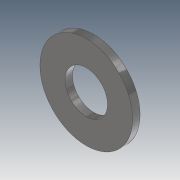
# Autodesk Inventor part: MCMASTER 92141A009
Saved by Autodesk Inventor 2020.4 (Build 244396000, 396)
## iProperties
RuleStatus: InUse
AfterDocSave0: file://Part Number Cleaner
Created: 2014-07-21
Material: STAINLESS STEEL, 18-8
Vendor: HHMI: JFRC - ID&F
Document SubType Name: Modeling
Designer: COOPB
Mass: 0.342993 g
Surface Area: 1.45791 cm^2
Volume: 0.0428742 cm^3
Density: 8 g/cm^3
Project: COMMON
Description: FLAT WASHER, #8
Appearance: Stainless - Brushed
LAB/DEPT: COMMON
REQUESTING SCIENTIST: COMMON
SURFACE ROUGHNESS: N/A
DESIGN DEPARTMENT: HHMI: JFRC - ID&F
SPECIAL FINISH: NONE
ALTERED ITEM PART NUMBER: N/A
ALTERED ITEM VENDOR: N/A
ALTERED ITEM DESCRIPTION: N/A
Author: COOPB
Revision Number: 0
Autodesk Inventor part; units mm, degrees
ref_plane "YZ Plane" through (0, 0, 0) normal (1, 0, 0) x (0, 1, 0)
ref_plane "XZ Plane" through (0, 0, 0) normal (0, 1, 0) x (-1, 0, 0)
ref_plane "XY Plane" through (0, 0, 0) normal (0, 0, 1) x (1, 0, 0)
sketch "Sketch1" plane through (0, 0, 0) normal (0, 0, 1) x (1, 0, 0)
  line L0 (0, 6.6675) -> (0, -6.6675) construction
  line L1 (-6.6675, 0) -> (6.6675, 0) construction
  circle A0 centre (0, 0) radius 4.7625
  circle A1 centre (0, 0) radius 2.1844
  dimension "d0" = 9.525
  dimension "d1" = 4.3688
  constraints: 2 centre point, 2 coincident
  measures "d0" diameter of A0
  measures "d1" diameter of A1
extrude "Extrusion1" add sketch "Sketch1" along normal blind 0.762
body "Solid1"
